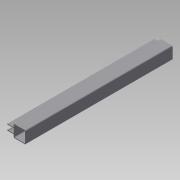
# Autodesk Inventor part: 9025
Saved by Autodesk Inventor 2013 (Build 170138000, 138)
## iProperties
Created: 2014-04-23
Part Number: 9025
Material: Generic
Document SubType Name: Modeling
Density: 1 g/cm^3
Vendor: 80/20 Inc.
Engineer: Ross Bowman
Designer: Ross Bowman
Catalog Web Link: 8020.net
Company: 80/20 Inc.
Author: Ross Bowman
Keywords: 80/20 , 8020 , T-Slot , Extrusion
Material: 6105-T5 Aluminum
Autodesk Inventor part; units mm, degrees
ref_plane "YZ Plane" through (0, 0, 0) normal (1, 0, 0) x (0, 1, 0)
ref_plane "XZ Plane" through (0, 0, 0) normal (0, 1, 0) x (-1, 0, 0)
ref_plane "XY Plane" through (0, 0, 0) normal (0, 0, 1) x (1, 0, 0)
sketch "Sketch1" plane through (0, 0, 0) normal (0, 0, 1) x (1, 0, 0)
  arc A0 (-11.176, -9.652) -> (-9.652, -11.176) centre (-9.652, -9.652) ccw
  line L0 (-11.176, 9.652) -> (-11.176, -9.652)
  arc A1 (-9.652, 11.176) -> (-11.176, 9.652) centre (-9.652, 9.652) ccw
  line L1 (9.652, 11.176) -> (-9.652, 11.176)
  arc A2 (11.176, 9.652) -> (9.652, 11.176) centre (9.652, 9.652) ccw
  line L2 (11.176, -9.652) -> (11.176, 9.652)
  arc A3 (9.652, -11.176) -> (11.176, -9.652) centre (9.652, -9.652) ccw
  line L3 (-9.652, -11.176) -> (9.652, -11.176)
  arc A4 (12.7, 10.5918) -> (10.5918, 12.7) centre (10.5918, 10.5918) ccw
  line L4 (10.5918, 12.7) -> (-10.5918, 12.7)
  arc A5 (-10.5918, 12.7) -> (-12.7, 10.5918) centre (-10.5918, 10.5918) ccw
  line L5 (-12.7, 10.5918) -> (-12.7, 6.731)
  arc A6 (-13.081, 6.35) -> (-12.7, 6.731) centre (-13.081, 6.731) ccw
  line L6 (-13.081, 6.35) -> (-25.019, 6.35)
  arc A7 (-25.019, 6.35) -> (-25.4, 5.969) centre (-25.019, 5.969) ccw
  line L7 (-25.4, 5.969) -> (-25.4, 4.826)
  arc A8 (-25.4, 4.826) -> (-24.638, 4.064) centre (-24.638, 4.826) ccw
  line L8 (-24.638, 4.064) -> (-23.0632, 4.064)
  arc A9 (-23.0632, 4.064) -> (-22.6822, 4.445) centre (-23.0632, 4.445) ccw
  arc A10 (-22.3012, 4.826) -> (-22.6822, 4.445) centre (-22.3012, 4.445) ccw
  line L9 (-22.3012, 4.826) -> (-13.081, 4.826)
  arc A11 (-12.7, 4.445) -> (-13.081, 4.826) centre (-13.081, 4.445) ccw
  line L10 (-12.7, 4.445) -> (-12.7, -4.445)
  arc A12 (-13.081, -4.826) -> (-12.7, -4.445) centre (-13.081, -4.445) ccw
  line L11 (-13.081, -4.826) -> (-22.3012, -4.826)
  arc A13 (-22.6822, -4.445) -> (-22.3012, -4.826) centre (-22.3012, -4.445) ccw
  arc A14 (-22.6822, -4.445) -> (-23.0632, -4.064) centre (-23.0632, -4.445) ccw
  line L12 (-23.0632, -4.064) -> (-24.638, -4.064)
  arc A15 (-24.638, -4.064) -> (-25.4, -4.826) centre (-24.638, -4.826) ccw
  line L13 (-25.4, -4.826) -> (-25.4, -5.969)
  arc A16 (-25.4, -5.969) -> (-25.019, -6.35) centre (-25.019, -5.969) ccw
  line L14 (-25.019, -6.35) -> (-13.081, -6.35)
  arc A17 (-12.7, -6.731) -> (-13.081, -6.35) centre (-13.081, -6.731) ccw
  line L15 (-12.7, -6.731) -> (-12.7, -10.5918)
  arc A18 (-12.7, -10.5918) -> (-10.5918, -12.7) centre (-10.5918, -10.5918) ccw
  line L16 (-10.5918, -12.7) -> (10.5918, -12.7)
  arc A19 (10.5918, -12.7) -> (12.7, -10.5918) centre (10.5918, -10.5918) ccw
  line L17 (12.7, -10.5918) -> (12.7, 10.5918)
  point P0 (0, 0)
  constraints: 40 point on circle, 38 tangent, 36 end point, 20 centre point, 13 parallel, 3 collinear, 1 horizontal, 1 vertical
extrude "Extrusion1" add sketch "Sketch1" against normal blind 304.8
body "Solid1"
